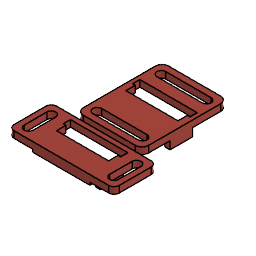
Gyroskop (Autodesk Fusion 360 design; units mm, degrees)
Autodesk Fusion 360 part; units mm, degrees
note: some values were not read from the file. Set by a fixed rule: which sketch regions a step uses.
sketch "Sketch1" plane through (0, 0, 0) normal (0, 0, 1) x (1, 0, 0)
  line L0 (0, 0) -> (20.5, 0)
  line L1 (20.5, 0) -> (20.5, 12)
  line L2 (20.5, 12) -> (0, 12)
  line L3 (0, 12) -> (0, 0)
  dimension "d1" = 20.5
  dimension "d2" = 12
  constraint horizontal L0
  constraint vertical L1
  constraint horizontal L2
  constraint vertical L3
  constraint coincident L0.start L3.end
  measures "d1" distance of L0.start L0.end
  measures "d2" distance of L0.start L2.end
extrude "Extrude1" add sketch "Sketch1" along normal blind 1.6 makes body 1
sketch "Sketch2" plane through (0, 0, 1.6) normal (0, 0, 1) x (-1, 0, 0)
  line L0 (0, -12) -> (0, 0)
  line L1 (0, 0) -> (-20.5, 0)
  line L2 (-20.5, 0) -> (-20.5, -12)
  line L3 (-20.5, -12) -> (0, -12)
  line L4 (-20.5, -12) -> (0, -12)
  line L5 (0, -12) -> (0, -9.5)
  line L6 (0, -9.5) -> (-20.5, -9.5)
  line L7 (-20.5, -9.5) -> (-20.5, -12)
  line L8 (0, -12) -> (-2.5, -12)
  line L9 (-2.5, -12) -> (-2.5, -9.5)
  line L10 (-2.5, -9.5) -> (0, -9.5)
  line L11 (0, -9.5) -> (0, -12)
  line L12 (-2.5714, -12) -> (-5.0714, -12)
  line L13 (-5.0714, -12) -> (-5.0714, -9.5)
  line L14 (-5.0714, -9.5) -> (-2.5714, -9.5)
  line L15 (-2.5714, -9.5) -> (-2.5714, -12)
  line L16 (-5.1429, -12) -> (-7.6429, -12)
  line L17 (-7.6429, -12) -> (-7.6429, -9.5)
  line L18 (-7.6429, -9.5) -> (-5.1429, -9.5)
  line L19 (-5.1429, -9.5) -> (-5.1429, -12)
  line L20 (-7.7143, -12) -> (-10.2143, -12)
  line L21 (-10.2143, -12) -> (-10.2143, -9.5)
  line L22 (-10.2143, -9.5) -> (-7.7143, -9.5)
  line L23 (-7.7143, -9.5) -> (-7.7143, -12)
  line L24 (-10.2857, -12) -> (-12.7857, -12)
  line L25 (-12.7857, -12) -> (-12.7857, -9.5)
  line L26 (-12.7857, -9.5) -> (-10.2857, -9.5)
  line L27 (-10.2857, -9.5) -> (-10.2857, -12)
  line L28 (-12.8571, -12) -> (-15.3571, -12)
  line L29 (-15.3571, -12) -> (-15.3571, -9.5)
  line L30 (-15.3571, -9.5) -> (-12.8571, -9.5)
  line L31 (-12.8571, -9.5) -> (-12.8571, -12)
  line L32 (-15.4286, -12) -> (-17.9286, -12)
  line L33 (-17.9286, -12) -> (-17.9286, -9.5)
  line L34 (-17.9286, -9.5) -> (-15.4286, -9.5)
  line L35 (-15.4286, -9.5) -> (-15.4286, -12)
  line L36 (-18, -12) -> (-20.5, -12)
  line L37 (-20.5, -12) -> (-20.5, -9.5)
  line L38 (-20.5, -9.5) -> (-18, -9.5)
  line L39 (-18, -9.5) -> (-18, -12)
  dimension "d9" = -18
  dimension "d10" = 0
  constraint horizontal L4
  constraint vertical L5
  constraint horizontal L6
  constraint vertical L7
  constraint coincident L0 L5.end
  constraint coincident L2.end L3.start
  constraint horizontal L8
  constraint vertical L9
  constraint horizontal L10
  constraint vertical L11
  constraint coincident L6 L9.end
extrude "Extrude2" add sketch "Sketch2" along normal blind 2.5 contours L0 L3 L4 L5 L6 L8 L9 L10 L11 | L3 L4 L6 L12 L13 L14 L15 | L2 L3 L4 L6 L7 L36 L37 L38 L39 | L3 L4 L6 L16 L17 L18 L19 | L3 L4 L6 L32 L33 L34 L35 | L3 L4 L6 L20 L21 L22 L23 | L3 L4 L6 L28 L29 L30 L31 | L3 L4 L6 L24 L25 L26 L27 bodies 1
sketch "Sketch3" plane through (0, 0, 4.1) normal (0, 0, 1) x (-1, 0, 0)
  line L0 (0, -9.5) -> (-2.5, -9.5)
  line L1 (-2.5, -9.5) -> (-2.5, -12)
  line L2 (-2.5, -12) -> (0, -12)
  line L3 (0, -12) -> (0, -9.5)
  line L4 (-1, -11) -> (-1.5, -11)
  line L5 (-1.5, -11) -> (-1.5, -10.5)
  line L6 (-1.5, -10.5) -> (-1, -10.5)
  line L7 (-1, -10.5) -> (-1, -11)
  line L8 (-3.5714, -10.5) -> (-3.5714, -11)
  line L9 (-3.5714, -11) -> (-4.0714, -11)
  line L10 (-4.0714, -11) -> (-4.0714, -10.5)
  line L11 (-4.0714, -10.5) -> (-3.5714, -10.5)
  line L12 (-6.1429, -10.5) -> (-6.1429, -11)
  line L13 (-6.1429, -11) -> (-6.6429, -11)
  line L14 (-6.6429, -11) -> (-6.6429, -10.5)
  line L15 (-6.6429, -10.5) -> (-6.1429, -10.5)
  line L16 (-8.7143, -10.5) -> (-8.7143, -11)
  line L17 (-8.7143, -11) -> (-9.2143, -11)
  line L18 (-9.2143, -11) -> (-9.2143, -10.5)
  line L19 (-9.2143, -10.5) -> (-8.7143, -10.5)
  line L20 (-11.2857, -10.5) -> (-11.2857, -11)
  line L21 (-11.2857, -11) -> (-11.7857, -11)
  line L22 (-11.7857, -11) -> (-11.7857, -10.5)
  line L23 (-11.7857, -10.5) -> (-11.2857, -10.5)
  line L24 (-13.8571, -10.5) -> (-13.8571, -11)
  line L25 (-13.8571, -11) -> (-14.3571, -11)
  line L26 (-14.3571, -11) -> (-14.3571, -10.5)
  line L27 (-14.3571, -10.5) -> (-13.8571, -10.5)
  line L28 (-16.4286, -10.5) -> (-16.4286, -11)
  line L29 (-16.4286, -11) -> (-16.9286, -11)
  line L30 (-16.9286, -11) -> (-16.9286, -10.5)
  line L31 (-16.9286, -10.5) -> (-16.4286, -10.5)
  line L32 (-19, -10.5) -> (-19, -11)
  line L33 (-19, -11) -> (-19.5, -11)
  line L34 (-19.5, -11) -> (-19.5, -10.5)
  line L35 (-19.5, -10.5) -> (-19, -10.5)
  dimension "d13" = -18
  dimension "d14" = 0
  constraint horizontal L4
  constraint vertical L5
  constraint horizontal L6
  constraint vertical L7
extrude "Extrude3" add sketch "Sketch3" along normal blind 6 contours L4 L5 L6 L7 | L8 L9 L10 L11 | L12 L13 L14 L15 | L16 L17 L18 L19 | L20 L21 L22 L23 | L24 L25 L26 L27 | L28 L29 L30 L31 | L32 L33 L34 L35 bodies 1
fillet "Fillet1" radius 0.1 32 edges at (18, 9.5, 2.85) (17.9286, 9.5, 2.85) (15.4286, 9.5, 2.85) (15.3571, 9.5, 2.85) (12.8571, 9.5, 2.85) (12.7857, 9.5, 2.85) (10.2857, 9.5, 2.85) (10.2143, 9.5, 2.85) (7.7143, 9.5, 2.85) (7.6429, 9.5, 2.85) (5.1429, 9.5, 2.85) (5.0714, 9.5, 2.85) (2.5714, 9.5, 2.85) (2.5, 9.5, 2.85) (0, 9.5, 2.85) (0, 12, 2.05) (2.5, 12, 2.85) (2.5714, 12, 2.85) (5.0714, 12, 2.85) (5.1429, 12, 2.85) (7.6429, 12, 2.85) (7.7143, 12, 2.85) (10.2143, 12, 2.85) (10.2857, 12, 2.85) (12.7857, 12, 2.85) (12.8571, 12, 2.85) (15.3571, 12, 2.85) (15.4286, 12, 2.85) (17.9286, 12, 2.85) (18, 12, 2.85) (20.5, 12, 2.05) (20.5, 9.5, 2.85) on bodies 1
sketch "Sketch4" plane through (0, 0, 0) normal (0, 0, -1) x (1, 0, 0)
  arc A0 (20.4, -12) -> (20.5, -11.9) centre (20.4, -11.9) ccw
  line L0 (20.5, -11.9) -> (20.5, 0)
  line L1 (20.5, 0) -> (0, 0)
  line L2 (0, 0) -> (0, -11.9)
  arc A1 (0, -11.9) -> (0.1, -12) centre (0.1, -11.9) ccw
  line L3 (0.1, -12) -> (20.4, -12)
  line L4 (7.5, -3) -> (13, -3)
  line L5 (13, -3) -> (13, -7)
  line L6 (13, -7) -> (7.5, -7)
  line L7 (7.5, -7) -> (7.5, -3)
  line L8 (0.5, -2) -> (1.5, -2)
  line L9 (1.5, -2) -> (1.5, -4)
  line L10 (1.5, -4) -> (0.5, -4)
  line L11 (0.5, -4) -> (0.5, -2)
  line L12 (2.5, -4) -> (2.5, -2)
  line L13 (2.5, -2) -> (3.5, -2)
  line L14 (3.5, -2) -> (3.5, -4)
  line L15 (3.5, -4) -> (2.5, -4)
  line L16 (14, -8.5) -> (14, -6.5)
  line L17 (14, -6.5) -> (15, -6.5)
  line L18 (15, -6.5) -> (15, -8.5)
  line L19 (15, -8.5) -> (14, -8.5)
  line L20 (17, -6.5) -> (17, -8.5)
  line L21 (17, -8.5) -> (16, -8.5)
  line L22 (16, -6.5) -> (17, -6.5)
  line L23 (16, -8.5) -> (16, -6.5)
  line L24 (6.5, -2.5) -> (4.5, -2.5)
  line L25 (4.5, -2.5) -> (4.5, -1.5)
  line L26 (4.5, -1.5) -> (6.5, -1.5)
  line L27 (6.5, -1.5) -> (6.5, -2.5)
  line L28 (6.5, -4) -> (4.5, -4)
  line L29 (4.5, -4) -> (4.5, -3)
  line L30 (6.5, -3) -> (6.5, -4)
  line L31 (4.5, -3) -> (6.5, -3)
  line L32 (4.5, -5) -> (6.5, -5)
  line L33 (6.5, -5) -> (6.5, -6)
  line L34 (6.5, -6) -> (4.5, -6)
  line L35 (4.5, -6) -> (4.5, -5)
  line L36 (6.5, -7.5) -> (4.5, -7.5)
  line L37 (4.5, -7.5) -> (4.5, -6.5)
  line L38 (6.5, -6.5) -> (6.5, -7.5)
  line L39 (4.5, -6.5) -> (6.5, -6.5)
  line L40 (6.5, -9) -> (4.5, -9)
  line L41 (4.5, -9) -> (4.5, -8)
  line L42 (4.5, -8) -> (6.5, -8)
  line L43 (6.5, -8) -> (6.5, -9)
  line L44 (15.5, -4) -> (15.5, -3)
  line L45 (15.5, -3) -> (17.5, -3)
  line L46 (17.5, -3) -> (17.5, -4)
  line L47 (17.5, -4) -> (15.5, -4)
  line L48 (15.5, -2.5) -> (15.5, -1.5)
  line L49 (15.5, -1.5) -> (17.5, -1.5)
  line L50 (17.5, -2.5) -> (15.5, -2.5)
  line L51 (17.5, -1.5) -> (17.5, -2.5)
  line L52 (13.5, -5) -> (15.5, -5)
  line L53 (15.5, -5) -> (15.5, -6)
  line L54 (15.5, -6) -> (13.5, -6)
  line L55 (13.5, -6) -> (13.5, -5)
  line L56 (18, -6) -> (16, -6)
  line L57 (16, -6) -> (16, -5)
  line L58 (16, -5) -> (18, -5)
  line L59 (18, -5) -> (18, -6)
  line L60 (7.5, -1.5) -> (13.5, -1.5)
  line L61 (13.5, -1.5) -> (13.5, -2.5)
  line L62 (13.5, -2.5) -> (7.5, -2.5)
  line L63 (7.5, -2.5) -> (7.5, -1.5)
  dimension "d19" = 5.5
  dimension "d20" = 4
  constraint horizontal L4
  constraint vertical L5
  constraint horizontal L6
  constraint vertical L7
  constraint horizontal L8
  constraint vertical L9
  constraint horizontal L10
  constraint vertical L11
  constraint horizontal L13
  constraint vertical L14
  constraint horizontal L15
  constraint vertical L12
  constraint horizontal L17
  constraint vertical L18
  constraint horizontal L19
  constraint vertical L16
  constraint horizontal L22
  constraint vertical L20
  constraint horizontal L21
  constraint vertical L23
  constraint horizontal L60
  constraint vertical L61
  constraint horizontal L62
  constraint vertical L63
  measures "d19" distance of L4.start L4.end
  measures "d20" distance of L4.start L6.end
extrude "Extrude4" add sketch "Sketch4" along normal blind 0.5 contours L8 L9 L10 L11 | L12 L13 L14 L15 | L16 L17 L18 L19 | L20 L21 L22 L23 | L24 L25 L26 L27 | L28 L29 L30 L31 | L32 L33 L34 L35 | L36 L37 L38 L39 | L40 L41 L42 L43 | L44 L45 L46 L47 | L48 L49 L50 L51 | L52 L53 L54 L55 | L56 L57 L58 L59 bodies 1
extrude "Extrude5" add sketch "Sketch4" along normal blind 1 contours L4 L5 L6 L7 | L60 L61 L62 L63 bodies 1
sketch "Sketch7" plane through (0, 0, 0) normal (0, 0, -1) x (1, 0, 0)
  circle A0 centre (1.25, -10.75) radius 0.7906
  circle A1 centre (3.8214, -10.75) radius 0.7906
  circle A2 centre (6.3929, -10.75) radius 0.7906
  circle A3 centre (8.9643, -10.75) radius 0.7906
  circle A4 centre (11.5357, -10.75) radius 0.7906
  circle A5 centre (14.1071, -10.75) radius 0.7906
  circle A6 centre (16.6786, -10.75) radius 0.7906
  circle A7 centre (19.25, -10.75) radius 0.7906
  dimension "d27" = 18
  dimension "d28" = 0
extrude "Extrude6" add sketch "Sketch7" along normal blind 0.5 bodies 1
chamfer "Chamfer1" distance 0.5 angle 45 8 edges at (0.5129, 11.0359, -0.5) (3.0844, 11.0359, -0.5) (5.6558, 11.0359, -0.5) (8.2272, 11.0359, -0.5) (10.7986, 11.0359, -0.5) (13.3701, 11.0359, -0.5) (15.9415, 11.0359, -0.5) (18.5129, 11.0359, -0.5) on bodies 1
sketch "Sketch8" plane through (0, 0, 0) normal (0, 0, 1) x (1, 0, 0)
  line L0 (22.5, 14) -> (-2, 14)
  line L1 (-2, 14) -> (-2, -2)
  line L2 (-2, -2) -> (22.5, -2)
  line L3 (22.5, -2) -> (22.5, 14)
  line L4 (21, 12.5) -> (-0.5, 12.5)
  line L5 (-0.5, 12.5) -> (-0.5, 9.5)
  line L6 (21, 9.5) -> (21, 12.5)
  line L7 (0.5, 9.5) -> (0.5, 6)
  line L8 (21, 9.5) -> (20, 9.5)
  line L9 (20, 9.5) -> (20, 6)
  line L10 (20, 6) -> (0.5, 6)
  line L11 (0.5, 6) -> (0.5, 9.5)
  line L12 (20, 9.5) -> (20, 6)
  line L13 (-0.5, 9.5) -> (0.5, 9.5)
  line L14 (20, 9.5) -> (21, 9.5)
  dimension "d68" = 1
  dimension "d69" = 1
  constraint horizontal L0
  constraint vertical L1
  constraint horizontal L2
  constraint vertical L3
  constraint horizontal L4
  constraint vertical L5
  constraint horizontal L13
  constraint vertical L6
  constraint vertical L7
  constraint horizontal L8
  constraint vertical L9
  constraint horizontal L10
  constraint vertical L11
  constraint vertical L12
  constraint coincident L9 L10.start
  constraint collinear L13 L14
  measures "d68" distance of L6.start L8.end
  measures "d69" distance of L5.end L7.start
extrude "Extrude7" add sketch "Sketch8" along normal blind 2.5 separate body makes body 2
move_body "Move1" bodies 1 to x (1, 0, 0) y (0, 1, 0) z (0, 0, 1) at (0, 0.2, -1.7)
sketch "Sketch9" plane through (0, 0, 0) normal (0, 0, -1) x (1, 0, 0)
  line L0 (22.5, -14) -> (22.5, 2)
  line L1 (22.5, 2) -> (-2, 2)
  line L2 (-2, 2) -> (-2, -14)
  line L3 (-2, -14) -> (22.5, -14)
  line L4 (-2, -9) -> (-0.2, -9)
  line L5 (-0.2, -9) -> (-0.2, -0.5)
  line L6 (-0.2, -0.5) -> (-2, -0.5)
  line L7 (-2, -0.5) -> (-2, -9)
  line L8 (10.25, -14) -> (10.25, 2) construction
  line L9 (20.7, -0.5) -> (22.5, -0.5)
  line L10 (22.5, -0.5) -> (22.5, -9)
  line L11 (22.5, -9) -> (20.7, -9)
  line L12 (20.7, -9) -> (20.7, -0.5)
  line L13 (20, -6) -> (20, -9.5)
  line L14 (20, -9.5) -> (21, -9.5)
  line L15 (21, -9.5) -> (21, -12.5)
  line L16 (21, -12.5) -> (-0.5, -12.5)
  line L17 (-0.5, -12.5) -> (-0.5, -9.5)
  line L18 (-0.5, -9.5) -> (0.5, -9.5)
  line L19 (0.5, -9.5) -> (0.5, -6)
  line L20 (0.5, -6) -> (20, -6)
  dimension "d34" = 1.8
  constraint horizontal L4
  constraint vertical L5
  constraint horizontal L6
  constraint vertical L7
  constraint coincident L2 L4.start
  constraint midpoint L3 L8.start
  constraint midpoint L1 L8.end
  constraint symmetric L4.start L8 L10.end
  constraint symmetric L4.end L8 L11.end
  constraint symmetric L5.end L8 L9.start
  constraint symmetric L6.end L8 L9.end
  measures "d34" distance of L4.start L4.end
extrude "Extrude8" add sketch "Sketch9" along normal blind 3 contours L0 L9 L10 L11 L12 | L2 L4 L5 L6 L7 bodies 2
sketch "Sketch10" plane through (0, 0.5, 0) normal (0, -1, 0) x (1, 0, 0)
  line L0 (-0.2, 0) -> (-2, 0)
  line L1 (-2, 0) -> (-2, -3)
  line L2 (-2, -3) -> (-0.2, -3)
  line L3 (-0.2, -3) -> (-0.2, 0)
  line L4 (-0.2, -3) -> (-0.19, -3)
  line L5 (-0.2, -1.5) -> (-0.2, -1.75)
  line L6 (-0.2, -1.75) -> (0.4, -1.75)
  line L7 (0.4, -1.75) -> (-0.19, -3)
  line L8 (-0.2, -1.75) -> (20.7, -1.75) construction
  line L9 (10.25, -1.75) -> (10.25, -4.737) construction
  line L10 (20.7, -1.5) -> (20.7, -1.75)
  line L11 (20.7, -1.75) -> (20.1, -1.75)
  line L12 (20.1, -1.75) -> (20.69, -3)
  line L13 (20.7, -3) -> (20.69, -3)
  line L14 (-0.2, -3) -> (-0.2, -1.75)
  line L15 (20.7, -3) -> (20.7, -1.75)
  dimension "d37" = 0.25
  dimension "d38" = 0.6
  dimension "d41" = 20.9
  constraint coincident L2.end L3.start
  constraint perpendicular L3 L4
  constraint midpoint L3 L5.start
  constraint parallel L3 L5
  constraint perpendicular L3 L6
  constraint perpendicular L5 L8
  constraint midpoint L8 L9.start
  constraint perpendicular L8 L9
  constraint symmetric L2.end L9 L13.start
  constraint symmetric L4.end L9 L12.end
  constraint symmetric L5.start L9 L10.start
  constraint symmetric L5.end L9 L8.end
  constraint symmetric L6.end L9 L11.end
  measures "d37" distance of L5.start L5.end
  measures "d38" distance of L5.end L6.end
  measures "d41" distance of L5.end L8.end
extrude "Extrude9" add sketch "Sketch10" against normal blind 8.5 contours L3 L4 L6 L7 L14 | L11 L12 L13 L15 bodies 2
extrude "Extrude18" add 1 faces at (13.8333, 12.5, 1.6667) along direction (0, -1, 0) blind 0.3 on bodies 2 bodies 2
copy_body "CopyPasteBodies1" bodies 2 makes body 3
sketch "Sketch11" plane through (0, 0, 0) normal (0, 0, -1) x (1, 0, 0)
  line L0 (-0.2, -9) -> (-2, -9)
  line L1 (-2, -9) -> (-2, -14)
  line L2 (-2, -14) -> (22.5, -14)
  line L3 (22.5, -14) -> (22.5, -9)
  line L4 (22.5, -9) -> (20.7, -9)
  line L5 (20.7, -9) -> (20.7, -0.5)
  line L6 (20.7, -0.5) -> (22.5, -0.5)
  line L7 (22.5, -0.5) -> (22.5, 2)
  line L8 (22.5, 2) -> (-2, 2)
  line L9 (-2, 2) -> (-2, -0.5)
  line L10 (-2, -0.5) -> (-0.2, -0.5)
  line L11 (-0.2, -0.5) -> (-0.2, -9)
  line L12 (22.5, -10.5) -> (-2, -10.5) construction
  line L13 (22.5, -14) -> (22.5, 2) construction
  line L14 (22.5, -14) -> (-2, -14) construction
  line L15 (-2, -14) -> (-2, 2) construction
  line L16 (-2, 2) -> (22.5, 2) construction
  line L17 (22.5, 2) -> (22.5, -14) construction
  line L18 (22.5, -14) -> (28, -14)
  line L19 (30, -12) -> (30, 0)
  line L20 (28, 2) -> (22.5, 2)
  line L21 (22.5, 2) -> (22.5, -14)
  line L22 (10.25, -6) -> (26.25, -6) construction
  line L23 (24.6, -1.75) -> (24.6, -10.25)
  arc A0 (24.6, -10.25) -> (27.9, -10.25) centre (26.25, -10.25) ccw
  line L24 (27.9, -10.25) -> (27.9, -1.75)
  arc A1 (27.9, -1.75) -> (24.6, -1.75) centre (26.25, -1.75) ccw
  line L25 (26.25, -1.75) -> (26.25, -10.25) construction
  arc A2 (28, -14) -> (30, -12) centre (28, -12) ccw
  arc A3 (30, 0) -> (28, 2) centre (28, 0) ccw
  line L26 (10.25, -14) -> (10.25, 2) construction
  line L27 (-9.5, -12) -> (-9.5, 0)
  arc A4 (-7.5, 2) -> (-9.5, 0) centre (-7.5, 0) ccw
  line L28 (-7.5, 2) -> (-2, 2)
  line L29 (-2, 2) -> (-2, -14)
  arc A5 (-9.5, -12) -> (-7.5, -14) centre (-7.5, -12) ccw
  line L30 (-2, -14) -> (-7.5, -14)
  arc A6 (-4.1, -1.75) -> (-7.4, -1.75) centre (-5.75, -1.75) ccw
  line L31 (-4.1, -1.75) -> (-4.1, -10.25)
  line L32 (-7.4, -10.25) -> (-7.4, -1.75)
  arc A7 (-7.4, -10.25) -> (-4.1, -10.25) centre (-5.75, -10.25) ccw
  line L33 (20, -6) -> (20, -9.5)
  line L34 (20, -9.5) -> (21, -9.5)
  line L35 (21, -9.5) -> (21, -12.2)
  line L36 (-0.5, -12.2) -> (-0.5, -9.5)
  line L37 (0.5, -9.5) -> (0.5, -6)
  line L38 (0.5, -6) -> (20, -6)
  line L39 (21, -12.2) -> (-0.5, -12.2)
  line L40 (-0.5, -9.5) -> (0.5, -9.5)
  point P0 (26.25, -6)
  dimension "d42" = 24.5
  dimension "d43" = 16
  dimension "d44" = 3.3
  dimension "d45" = 8.5
  dimension "d46" = 2
  constraint coincident L3 L12.start
  constraint coincident L1 L12.end
  constraint perpendicular L1 L12
  constraint coincident L2.end L3.start
  constraint coincident L7.end L8.start
  constraint horizontal L14
  constraint vertical L15
  constraint horizontal L16
  constraint vertical L17
  constraint coincident L8.end L9.start
  constraint horizontal L18
  constraint vertical L19
  constraint horizontal L20
  constraint vertical L21
  constraint perpendicular L13 L22
  constraint tangent L23 A0
  constraint tangent A0 L24
  constraint parallel L23 L24
  constraint tangent L24 A1
  constraint tangent L23 A1
  constraint perpendicular L22 L25
  constraint coincident P0 L22.end
  constraint midpoint L25 P0
  constraint tangent L18 A2
  constraint tangent L19 A2
  constraint tangent L19 A3
  constraint tangent L20 A3
  constraint equal A2 A3
  constraint midpoint L14 L26.start
  constraint midpoint L16 L26.end
  constraint symmetric L2.end L26 L1.end
  constraint symmetric L7.end L26 L8.end
  constraint symmetric L23.start L26 A6.start
  constraint symmetric L23.end L26 L31.end
  constraint symmetric A0.end L26 L32.start
  constraint symmetric L24.end L26 A6.end
  constraint symmetric A0 L26 A7
  constraint symmetric A1 L26 A6
  constraint symmetric L18.end L26 A5.end
  constraint symmetric L19.start L26 L27.start
  constraint symmetric A2 L26 A5
  constraint symmetric L19.end L26 L27.end
  constraint symmetric L20.start L26 A4.start
  constraint symmetric A3 L26 A4
  measures "d42" distance of L13 L15
  measures "d43" distance of L22.start P0
  measures "d44" diameter of A0
  measures "d45" distance of A1.centre A0.centre
  measures "d46" radius of A2
extrude "Extrude10" add sketch "Sketch11" against normal blind 2.5 contours L1 L9 L27 A4 L28 L29 A5 L30 | L3 L7 L18 L19 L20 L21 A2 A3 bodies 2
sketch "Sketch12" plane through (0, 0, 0) normal (0, 0, -1) x (1, 0, 0)
  line L0 (-0.2, -9) -> (-2, -9)
  line L1 (-2, -9) -> (-2, -14)
  line L2 (-2, -14) -> (22.5, -14)
  line L3 (22.5, -14) -> (22.5, -9)
  line L4 (22.5, -9) -> (20.7, -9)
  line L5 (20.7, -9) -> (20.7, -0.5)
  line L6 (20.7, -0.5) -> (22.5, -0.5)
  line L7 (22.5, -0.5) -> (22.5, 2)
  line L8 (22.5, 2) -> (-2, 2)
  line L9 (-2, 2) -> (-2, -0.5)
  line L10 (-2, -0.5) -> (-0.2, -0.5)
  line L11 (-0.2, -0.5) -> (-0.2, -9)
  line L12 (10.25, -14) -> (10.25, 2) construction
  line L13 (22.5, -6) -> (-2, -6) construction
  line L14 (22.5, -14) -> (-2, -14) construction
  line L15 (-2, -14) -> (-2, 2) construction
  line L16 (-2, 2) -> (22.5, 2) construction
  line L17 (22.5, 2) -> (22.5, -14) construction
  line L18 (10.25, -6) -> (10.25, -18) construction
  line L19 (10.25, -18) -> (10.25, 6) construction
  line L20 (22.5, -14) -> (-2, -14)
  line L21 (-2, -14) -> (-2, -19.5)
  line L22 (0.5, -22) -> (20, -22)
  line L23 (22.5, -19.5) -> (22.5, -14)
  line L24 (18.75, -16.35) -> (1.75, -16.35)
  arc A0 (1.75, -16.35) -> (1.75, -19.65) centre (1.75, -18) ccw
  line L25 (1.75, -19.65) -> (18.75, -19.65)
  arc A1 (18.75, -19.65) -> (18.75, -16.35) centre (18.75, -18) ccw
  line L26 (18.75, -18) -> (1.75, -18) construction
  arc A2 (-2, -19.5) -> (0.5, -22) centre (0.5, -19.5) ccw
  arc A3 (20, -22) -> (22.5, -19.5) centre (20, -19.5) ccw
  line L27 (22.5, 7.5) -> (22.5, 2)
  line L28 (22.5, 2) -> (-2, 2)
  line L29 (-2, 2) -> (-2, 7.5)
  arc A4 (0.5, 10) -> (-2, 7.5) centre (0.5, 7.5) ccw
  line L30 (0.5, 10) -> (20, 10)
  arc A5 (22.5, 7.5) -> (20, 10) centre (20, 7.5) ccw
  line L31 (18.75, 4.35) -> (1.75, 4.35)
  arc A6 (1.75, 7.65) -> (1.75, 4.35) centre (1.75, 6) ccw
  arc A7 (18.75, 4.35) -> (18.75, 7.65) centre (18.75, 6) ccw
  line L32 (1.75, 7.65) -> (18.75, 7.65)
  line L33 (20, -6) -> (20, -9.5)
  line L34 (20, -9.5) -> (21, -9.5)
  line L35 (21, -9.5) -> (21, -12.2)
  line L36 (-0.5, -12.2) -> (-0.5, -9.5)
  line L37 (0.5, -9.5) -> (0.5, -6)
  line L38 (0.5, -6) -> (20, -6)
  line L39 (21, -12.2) -> (-0.5, -12.2)
  line L40 (-0.5, -9.5) -> (0.5, -9.5)
  point P0 (10.25, -18)
  dimension "d49" = 3.3
  dimension "d50" = 2.5
  dimension "d51" = 17
  constraint midpoint L2 L12.start
  constraint midpoint L8 L12.end
  constraint perpendicular L11 L13
  constraint horizontal L14
  constraint vertical L15
  constraint horizontal L16
  constraint vertical L17
  constraint coincident L8.end L9.start
  constraint coincident L2.end L3.start
  constraint midpoint L12 L18.start
  constraint perpendicular L2 L18
  constraint perpendicular L8 L19
  constraint horizontal L20
  constraint vertical L21
  constraint horizontal L22
  constraint vertical L23
  constraint tangent L24 A0
  constraint tangent A0 L25
  constraint parallel L24 L25
  constraint tangent L25 A1
  constraint tangent L24 A1
  constraint perpendicular L21 L26
  constraint coincident P0 L18.end
  constraint midpoint L26 P0
  constraint tangent L21 A2
  constraint tangent L22 A2
  constraint tangent L22 A3
  constraint tangent L23 A3
  constraint equal A2 A3
  constraint symmetric L13 L2.end L7.end
  constraint symmetric L13 L1.end L8.end
  constraint symmetric L13 L24.start L31.start
  constraint symmetric L13 L24.end L31.end
  constraint symmetric L13 A0.end A6.start
  constraint symmetric L13 L25.end A7.end
  constraint symmetric L13 A0 A6
  constraint symmetric L13 A1 A7
  constraint symmetric L13 L21.end L29.end
  constraint symmetric L13 L22.start A4.start
  constraint symmetric L13 A2 A4
  constraint symmetric L13 L22.end L30.end
  constraint symmetric L13 L23.start L27.start
  constraint symmetric L13 A3 A5
  measures "d49" diameter of A0
  measures "d50" radius of A2
  measures "d51" distance of A1.centre A0.centre
extrude "Extrude11" add sketch "Sketch12" against normal blind 2.5 contours L2 L20 L21 L22 L23 A2 A3 | L8 L27 L28 L29 A4 L30 A5 bodies 3
extrude "Extrude13" cut 1 faces at (20.7, 6.1667, -0.5833) along direction (1, 0, 0) blind 0.3 on bodies 3 bodies 2 3
sketch "Sketch13" plane through (0, 0, 0) normal (0, 0, -1) x (1, 0, 0)
  line L0 (21, -9) -> (21, -0.5)
  line L1 (21, -0.5) -> (22.5, -0.5)
  line L2 (22.5, -19.5) -> (22.5, -9)
  arc A0 (22.5, 7.5) -> (20, 10) centre (20, 7.5) ccw
  line L3 (20, 10) -> (0.5, 10)
  arc A1 (0.5, 10) -> (-2, 7.5) centre (0.5, 7.5) ccw
  line L4 (-2, -9) -> (-2, -19.5)
  line L5 (-2, -0.5) -> (-0.2, -0.5)
  arc A2 (18.75, 4.35) -> (18.75, 7.65) centre (18.75, 6) ccw
  line L6 (18.75, 4.35) -> (1.75, 4.35)
  arc A3 (1.75, 7.65) -> (1.75, 4.35) centre (1.75, 6) ccw
  line L7 (1.75, 7.65) -> (18.75, 7.65)
  line L8 (-0.5, 0) -> (21, 0)
  line L9 (21, 0) -> (21, 2)
  line L10 (21, 2) -> (-0.5, 2)
  line L11 (-0.5, 2) -> (-0.5, 0)
  line L12 (-0.5, 0) -> (-0.5, 2)
  line L13 (21, 0) -> (21, 2)
  line L14 (0.5, -6) -> (20, -6)
  line L15 (0.5, -9.5) -> (0.5, -6)
  line L16 (20, -6) -> (20, -9.5)
  line L17 (-0.2, -0.5) -> (-0.2, -9)
  arc A4 (18.75, -19.65) -> (18.75, -16.35) centre (18.75, -18) ccw
  line L18 (18.75, -19.65) -> (1.75, -19.65)
  arc A5 (1.75, -16.35) -> (1.75, -19.65) centre (1.75, -18) ccw
  line L19 (1.75, -16.35) -> (18.75, -16.35)
  line L20 (-0.2, -9) -> (-2, -9)
  arc A6 (-2, -19.5) -> (0.5, -22) centre (0.5, -19.5) ccw
  line L21 (0.5, -22) -> (20, -22)
  arc A7 (20, -22) -> (22.5, -19.5) centre (20, -19.5) ccw
  line L22 (22.5, -9) -> (21, -9)
  line L23 (22.5, -0.5) -> (22.5, 7.5)
  line L24 (-2, 7.5) -> (-2, -0.5)
  line L25 (20, -9.5) -> (21, -9.5)
  line L26 (21, -9.5) -> (21, -12.2)
  line L27 (21, -12.2) -> (-0.5, -12.2)
  line L28 (-0.5, -12.2) -> (-0.5, -9.5)
  line L29 (-0.5, -9.5) -> (0.5, -9.5)
  constraint horizontal L8
  constraint vertical L9
  constraint horizontal L10
  constraint vertical L11
  constraint vertical L12
  constraint vertical L13
extrude "Extrude16" add sketch "Sketch13" along normal blind 1 contours L8 L9 L10 L11 L12 L13 bodies 3
extrude "Extrude17" add sketch "Sketch13" along normal blind 1 contours L8 L9 L10 L11 L12 L13 bodies 2
move_body "Move2" bodies 3 to x (1, 0, 0) y (0, 1, 0) z (0, 0, 1) at (0, 26, 0)
hidden bodies 1
named bodies: "Gyroscope", "GyroscponeHolder1", "Holder1", "GyroscopeHolder2"
